Autodesk Inventor part; units mm, degrees
(part 2 of 6)
  line L449 (30.3134, 44.4626) -> (30.5187, 44.7625) construction
  line L450 (30.5187, 44.7625) -> (30.9923, 45.236) construction
  line L451 (30.9923, 45.236) -> (31.2921, 45.4412) construction
  line L452 (31.2921, 45.4412) -> (31.9491, 45.7133) construction
  line L453 (31.9491, 45.7133) -> (32.3063, 45.7803) construction
  line L454 (32.3063, 45.7803) -> (32.9761, 45.7803) construction
  line L455 (32.9761, 45.7803) -> (33.3332, 45.7133) construction
  line L456 (33.3332, 45.7133) -> (33.9902, 45.4412) construction
  line L457 (33.9902, 45.4412) -> (34.2901, 45.236) construction
  line L458 (34.2901, 45.236) -> (34.7637, 44.7625) construction
  line L459 (34.7637, 44.7625) -> (34.969, 44.4626) construction
  line L460 (34.969, 44.4626) -> (35.2413, 43.8054) construction
  line L461 (35.2413, 43.8054) -> (35.3082, 43.4482) construction
  line L462 (35.3082, 43.4482) -> (35.3082, 42.7784) construction
  line L463 (35.3082, 42.7784) -> (35.2413, 42.4212) construction
  line L464 (35.2413, 42.4212) -> (34.969, 41.764) construction
  line L465 (34.969, 41.764) -> (34.7638, 41.4641) construction
  line L466 (34.7638, 41.4641) -> (34.2901, 40.9905) construction
  line L467 (34.2901, 40.9905) -> (33.9903, 40.7853) construction
  line L468 (33.9903, 40.7853) -> (33.3332, 40.5132) construction
  line L469 (33.3332, 40.5132) -> (32.976, 40.4463) construction
  line L470 (32.976, 40.4463) -> (32.6412, 40.4463) construction
  circle A90 centre (-16.6963, 38.4758) radius 1.25
  circle A91 centre (15.3037, 6.4758) radius 1.25
  circle A92 centre (15.3037, 38.4758) radius 1.25
  circle A93 centre (-16.6963, 6.4758) radius 1.25
  arc A94 (39.458, -65.8975) -> (33.108, -59.5475) centre (33.108, -65.8975) ccw
  line L471 (33.108, -59.5475) -> (31.785, -59.5475)
  arc A95 (26.4124, -59.0625) -> (31.785, -59.5475) centre (31.785, -29.5475) ccw
  arc A96 (26.4124, -59.0625) -> (21.0398, -58.5775) centre (21.0398, -88.5775) ccw
  line L472 (21.0398, -58.5775) -> (-15.8645, -58.5775)
  arc A97 (-15.8645, -56.5775) -> (-15.8645, -58.5775) centre (-15.8645, -57.5775) ccw
  line L473 (-15.8645, -56.5775) -> (23.218, -56.5775)
  arc A98 (23.218, -56.5775) -> (23.218, -54.5775) centre (23.218, -55.5775) ccw
  line L474 (23.218, -54.5775) -> (-15.8645, -54.5775)
  arc A99 (-15.8645, -52.5775) -> (-15.8645, -54.5775) centre (-15.8645, -53.5775) ccw
  line L475 (-15.8645, -52.5775) -> (23.218, -52.5775)
  arc A100 (23.218, -52.5775) -> (23.218, -50.5775) centre (23.218, -51.5775) ccw
  line L476 (23.218, -50.5775) -> (-15.8645, -50.5775)
  arc A101 (-15.8645, -48.5775) -> (-15.8645, -50.5775) centre (-15.8645, -49.5775) ccw
  line L477 (-15.8645, -48.5775) -> (23.218, -48.5775)
  arc A102 (23.218, -48.5775) -> (23.218, -46.5775) centre (23.218, -47.5775) ccw
  line L478 (23.218, -46.5775) -> (-15.8645, -46.5775)
  arc A103 (-15.8645, -44.5775) -> (-15.8645, -46.5775) centre (-15.8645, -45.5775) ccw
  line L479 (-15.8645, -44.5775) -> (23.218, -44.5775)
  arc A104 (23.218, -44.5775) -> (23.218, -42.5775) centre (23.218, -43.5775) ccw
  line L480 (23.218, -42.5775) -> (-15.8645, -42.5775)
  arc A105 (-15.8645, -40.5775) -> (-15.8645, -42.5775) centre (-15.8645, -41.5775) ccw
  line L481 (-15.8645, -40.5775) -> (23.218, -40.5775)
  arc A106 (23.218, -40.5775) -> (23.218, -38.5775) centre (23.218, -39.5775) ccw
  line L482 (23.218, -38.5775) -> (-15.8645, -38.5775)
  arc A107 (-15.8645, -36.5775) -> (-15.8645, -38.5775) centre (-15.8645, -37.5775) ccw
  line L483 (-15.8645, -36.5775) -> (23.218, -36.5775)
  arc A108 (23.218, -36.5775) -> (23.218, -34.5775) centre (23.218, -35.5775) ccw
  line L484 (23.218, -34.5775) -> (-15.8645, -34.5775)
  arc A109 (-15.8645, -32.5775) -> (-15.8645, -34.5775) centre (-15.8645, -33.5775) ccw
  line L485 (-15.8645, -32.5775) -> (21.0398, -32.5775)
  arc A110 (21.0398, -32.5775) -> (26.4124, -32.0925) centre (21.0398, -2.5775) ccw
  arc A111 (31.785, -31.6075) -> (26.4124, -32.0925) centre (31.785, -61.6075) ccw
  line L486 (31.785, -31.6075) -> (33.743, -31.6075)
  arc A112 (33.743, -31.6075) -> (40.093, -25.2575) centre (33.743, -25.2575) ccw
  line L487 (40.093, -25.2575) -> (40.093, -19.225)
  arc A113 (40.093, -19.225) -> (38.5055, -17.6375) centre (38.5055, -19.225) ccw
  line L488 (38.5055, -17.6375) -> (-36.4245, -17.6375)
  arc A114 (-36.4245, -17.6375) -> (-38.012, -19.225) centre (-36.4245, -19.225) ccw
  line L489 (-38.012, -19.225) -> (-38.012, -71.9264)
  arc A115 (-38.012, -71.9264) -> (-36.4245, -73.5139) centre (-36.4245, -71.9264) ccw
  line L490 (-36.4245, -73.5139) -> (37.8705, -73.5139)
  arc A116 (37.8705, -73.5139) -> (39.458, -71.9264) centre (37.8705, -71.9264) ccw
  line L491 (39.458, -71.9264) -> (39.458, -65.8975)
  spline S16 degree 3 poles (-31.027, -27.607) (-31.3618, -27.607) (-31.719, -27.5401) (-32.376, -27.2679) (-32.6759, -27.0627) (-33.1495, -26.5892) (-33.3548, -26.2892) (-33.627, -25.6321) (-33.694, -25.2748) (-33.694, -24.6051) (-33.627, -24.2478) (-33.3548, -23.5907) (-33.1495, -23.2907) (-32.6759, -22.8172) (-32.376, -22.612) (-31.719, -22.3399) (-31.3618, -22.273) (-30.6921, -22.273) (-30.3349, -22.3399) (-29.6779, -22.612) (-29.3781, -22.8172) (-28.9044, -23.2907) (-28.6991, -23.5907) (-28.4269, -24.2478) (-28.36, -24.6051) (-28.36, -25.2748) (-28.4269, -25.6321) (-28.6991, -26.2892) (-28.9044, -26.5892) (-29.378, -27.0627) (-29.6779, -27.2679) (-30.3349, -27.5401) (-30.6921, -27.607) (-31.027, -27.607) knots -1.607821 -1.607821 -1.607821 -1.607821 -1.507362 -1.507362 -1.406903 -1.406903 -1.30639 -1.30639 -1.205878 -1.205878 -1.105355 -1.105355 -1.004831 -1.004831 -0.904371 -0.904371 -0.803911 -0.803911 -0.70345 -0.70345 -0.60299 -0.60299 -0.502467 -0.502467 -0.401943 -0.401943 -0.301431 -0.301431 -0.200918 -0.200918 -0.100459 -0.100459 0 0 0 0
  line L492 (-31.027, -27.607) -> (-31.3618, -27.607) construction
  line L493 (-31.3618, -27.607) -> (-31.719, -27.5401) construction
  line L494 (-31.719, -27.5401) -> (-32.376, -27.2679) construction
  line L495 (-32.376, -27.2679) -> (-32.6759, -27.0627) construction
  line L496 (-32.6759, -27.0627) -> (-33.1495, -26.5892) construction
  line L497 (-33.1495, -26.5892) -> (-33.3548, -26.2892) construction
  line L498 (-33.3548, -26.2892) -> (-33.627, -25.6321) construction
  line L499 (-33.627, -25.6321) -> (-33.694, -25.2748) construction
  line L500 (-33.694, -25.2748) -> (-33.694, -24.6051) construction
  line L501 (-33.694, -24.6051) -> (-33.627, -24.2478) construction
  line L502 (-33.627, -24.2478) -> (-33.3548, -23.5907) construction
  line L503 (-33.3548, -23.5907) -> (-33.1495, -23.2907) construction
  line L504 (-33.1495, -23.2907) -> (-32.6759, -22.8172) construction
  line L505 (-32.6759, -22.8172) -> (-32.376, -22.612) construction
  line L506 (-32.376, -22.612) -> (-31.719, -22.3399) construction
  line L507 (-31.719, -22.3399) -> (-31.3618, -22.273) construction
  line L508 (-31.3618, -22.273) -> (-30.6921, -22.273) construction
  line L509 (-30.6921, -22.273) -> (-30.3349, -22.3399) construction
  line L510 (-30.3349, -22.3399) -> (-29.6779, -22.612) construction
  line L511 (-29.6779, -22.612) -> (-29.3781, -22.8172) construction
  line L512 (-29.3781, -22.8172) -> (-28.9044, -23.2907) construction
  line L513 (-28.9044, -23.2907) -> (-28.6991, -23.5907) construction
  line L514 (-28.6991, -23.5907) -> (-28.4269, -24.2478) construction
  line L515 (-28.4269, -24.2478) -> (-28.36, -24.6051) construction
  line L516 (-28.36, -24.6051) -> (-28.36, -25.2748) construction
  line L517 (-28.36, -25.2748) -> (-28.4269, -25.6321) construction
  line L518 (-28.4269, -25.6321) -> (-28.6991, -26.2892) construction
  line L519 (-28.6991, -26.2892) -> (-28.9044, -26.5892) construction
  line L520 (-28.9044, -26.5892) -> (-29.378, -27.0627) construction
  line L521 (-29.378, -27.0627) -> (-29.6779, -27.2679) construction
  line L522 (-29.6779, -27.2679) -> (-30.3349, -27.5401) construction
  line L523 (-30.3349, -27.5401) -> (-30.6921, -27.607) construction
  line L524 (-30.6921, -27.607) -> (-31.027, -27.607) construction
  spline S17 degree 3 poles (-31.027, -68.882) (-31.3618, -68.882) (-31.719, -68.8151) (-32.376, -68.5429) (-32.6759, -68.3377) (-33.1495, -67.8642) (-33.3548, -67.5643) (-33.627, -66.9071) (-33.694, -66.5499) (-33.694, -65.8801) (-33.627, -65.5229) (-33.3548, -64.8657) (-33.1495, -64.5658) (-32.6759, -64.0922) (-32.376, -63.887) (-31.719, -63.6149) (-31.3618, -63.548) (-30.6921, -63.548) (-30.3349, -63.6149) (-29.6779, -63.887) (-29.378, -64.0922) (-28.9044, -64.5658) (-28.6991, -64.8657) (-28.4269, -65.5229) (-28.36, -65.8801) (-28.36, -66.5499) (-28.4269, -66.9071) (-28.6991, -67.5643) (-28.9044, -67.8642) (-29.3781, -68.3377) (-29.6779, -68.5429) (-30.3349, -68.8151) (-30.6921, -68.882) (-31.027, -68.882) knots -1.607821 -1.607821 -1.607821 -1.607821 -1.507361 -1.507361 -1.406901 -1.406901 -1.306377 -1.306377 -1.205854 -1.205854 -1.105342 -1.105342 -1.004829 -1.004829 -0.90437 -0.90437 -0.803911 -0.803911 -0.703451 -0.703451 -0.602992 -0.602992 -0.50248 -0.50248 -0.401967 -0.401967 -0.301444 -0.301444 -0.200921 -0.200921 -0.10046 -0.10046 0 0 0 0
  line L525 (-31.027, -68.882) -> (-31.3618, -68.882) construction
  line L526 (-31.3618, -68.882) -> (-31.719, -68.8151) construction
  line L527 (-31.719, -68.8151) -> (-32.376, -68.5429) construction
  line L528 (-32.376, -68.5429) -> (-32.6759, -68.3377) construction
  line L529 (-32.6759, -68.3377) -> (-33.1495, -67.8642) construction
  line L530 (-33.1495, -67.8642) -> (-33.3548, -67.5643) construction
  line L531 (-33.3548, -67.5643) -> (-33.627, -66.9071) construction
  line L532 (-33.627, -66.9071) -> (-33.694, -66.5499) construction
  line L533 (-33.694, -66.5499) -> (-33.694, -65.8801) construction
  line L534 (-33.694, -65.8801) -> (-33.627, -65.5229) construction
  line L535 (-33.627, -65.5229) -> (-33.3548, -64.8657) construction
  line L536 (-33.3548, -64.8657) -> (-33.1495, -64.5658) construction
  line L537 (-33.1495, -64.5658) -> (-32.6759, -64.0922) construction
  line L538 (-32.6759, -64.0922) -> (-32.376, -63.887) construction
  line L539 (-32.376, -63.887) -> (-31.719, -63.6149) construction
  line L540 (-31.719, -63.6149) -> (-31.3618, -63.548) construction
  line L541 (-31.3618, -63.548) -> (-30.6921, -63.548) construction
  line L542 (-30.6921, -63.548) -> (-30.3349, -63.6149) construction
  line L543 (-30.3349, -63.6149) -> (-29.6779, -63.887) construction
  line L544 (-29.6779, -63.887) -> (-29.378, -64.0922) construction
  line L545 (-29.378, -64.0922) -> (-28.9044, -64.5658) construction
  line L546 (-28.9044, -64.5658) -> (-28.6991, -64.8657) construction
  line L547 (-28.6991, -64.8657) -> (-28.4269, -65.5229) construction
  line L548 (-28.4269, -65.5229) -> (-28.36, -65.8801) construction
  line L549 (-28.36, -65.8801) -> (-28.36, -66.5499) construction
  line L550 (-28.36, -66.5499) -> (-28.4269, -66.9071) construction
  line L551 (-28.4269, -66.9071) -> (-28.6991, -67.5643) construction
  line L552 (-28.6991, -67.5643) -> (-28.9044, -67.8642) construction
  line L553 (-28.9044, -67.8642) -> (-29.3781, -68.3377) construction
  line L554 (-29.3781, -68.3377) -> (-29.6779, -68.5429) construction
  line L555 (-29.6779, -68.5429) -> (-30.3349, -68.8151) construction
  line L556 (-30.3349, -68.8151) -> (-30.6921, -68.882) construction
  line L557 (-30.6921, -68.882) -> (-31.027, -68.882) construction
  spline S18 degree 3 poles (32.473, -68.882) (32.1382, -68.882) (31.781, -68.8151) (31.124, -68.5429) (30.8241, -68.3377) (30.3505, -67.8642) (30.1452, -67.5643) (29.873, -66.9071) (29.806, -66.5499) (29.806, -65.8801) (29.873, -65.5229) (30.1452, -64.8657) (30.3505, -64.5658) (30.8241, -64.0922) (31.124, -63.887) (31.781, -63.6149) (32.1382, -63.548) (32.8079, -63.548) (33.1651, -63.6149) (33.8221, -63.887) (34.122, -64.0922) (34.5956, -64.5658) (34.8009, -64.8657) (35.0731, -65.5229) (35.14, -65.8801) (35.14, -66.5499) (35.0731, -66.9071) (34.8009, -67.5643) (34.5956, -67.8642) (34.1219, -68.3377) (33.8221, -68.5429) (33.1651, -68.8151) (32.8079, -68.882) (32.473, -68.882) knots -1.607821 -1.607821 -1.607821 -1.607821 -1.507361 -1.507361 -1.406901 -1.406901 -1.306377 -1.306377 -1.205854 -1.205854 -1.105342 -1.105342 -1.004829 -1.004829 -0.90437 -0.90437 -0.803911 -0.803911 -0.703451 -0.703451 -0.602992 -0.602992 -0.50248 -0.50248 -0.401967 -0.401967 -0.301444 -0.301444 -0.200921 -0.200921 -0.10046 -0.10046 0 0 0 0
  line L558 (32.473, -68.882) -> (32.1382, -68.882) construction
  line L559 (32.1382, -68.882) -> (31.781, -68.8151) construction
  line L560 (31.781, -68.8151) -> (31.124, -68.5429) construction
  line L561 (31.124, -68.5429) -> (30.8241, -68.3377) construction
  line L562 (30.8241, -68.3377) -> (30.3505, -67.8642) construction
  line L563 (30.3505, -67.8642) -> (30.1452, -67.5643) construction
  line L564 (30.1452, -67.5643) -> (29.873, -66.9071) construction
  line L565 (29.873, -66.9071) -> (29.806, -66.5499) construction
  line L566 (29.806, -66.5499) -> (29.806, -65.8801) construction
  line L567 (29.806, -65.8801) -> (29.873, -65.5229) construction
  line L568 (29.873, -65.5229) -> (30.1452, -64.8657) construction
  line L569 (30.1452, -64.8657) -> (30.3505, -64.5658) construction
  line L570 (30.3505, -64.5658) -> (30.8241, -64.0922) construction
  line L571 (30.8241, -64.0922) -> (31.124, -63.887) construction
  line L572 (31.124, -63.887) -> (31.781, -63.6149) construction
  line L573 (31.781, -63.6149) -> (32.1382, -63.548) construction
  line L574 (32.1382, -63.548) -> (32.8079, -63.548) construction
  line L575 (32.8079, -63.548) -> (33.1651, -63.6149) construction
  line L576 (33.1651, -63.6149) -> (33.8221, -63.887) construction
  line L577 (33.8221, -63.887) -> (34.122, -64.0922) construction
  line L578 (34.122, -64.0922) -> (34.5956, -64.5658) construction
  line L579 (34.5956, -64.5658) -> (34.8009, -64.8657) construction
  line L580 (34.8009, -64.8657) -> (35.0731, -65.5229) construction
  line L581 (35.0731, -65.5229) -> (35.14, -65.8801) construction
  line L582 (35.14, -65.8801) -> (35.14, -66.5499) construction
  line L583 (35.14, -66.5499) -> (35.0731, -66.9071) construction
  line L584 (35.0731, -66.9071) -> (34.8009, -67.5643) construction
  line L585 (34.8009, -67.5643) -> (34.5956, -67.8642) construction
  line L586 (34.5956, -67.8642) -> (34.1219, -68.3377) construction
  line L587 (34.1219, -68.3377) -> (33.8221, -68.5429) construction
  line L588 (33.8221, -68.5429) -> (33.1651, -68.8151) construction
  line L589 (33.1651, -68.8151) -> (32.8079, -68.882) construction
  line L590 (32.8079, -68.882) -> (32.473, -68.882) construction
  spline S19 degree 3 poles (32.473, -27.607) (32.1382, -27.607) (31.781, -27.5401) (31.124, -27.2679) (30.8241, -27.0627) (30.3505, -26.5892) (30.1452, -26.2892) (29.873, -25.6321) (29.806, -25.2748) (29.806, -24.6051) (29.873, -24.2478) (30.1452, -23.5907) (30.3505, -23.2907) (30.8241, -22.8172) (31.124, -22.612) (31.781, -22.3399) (32.1382, -22.273) (32.8079, -22.273) (33.1651, -22.3399) (33.8221, -22.612) (34.1219, -22.8172) (34.5956, -23.2907) (34.8009, -23.5907) (35.0731, -24.2478) (35.14, -24.6051) (35.14, -25.2748) (35.0731, -25.6321) (34.8009, -26.2892) (34.5956, -26.5892) (34.122, -27.0627) (33.8221, -27.2679) (33.1651, -27.5401) (32.8079, -27.607) (32.473, -27.607) knots -1.607821 -1.607821 -1.607821 -1.607821 -1.507362 -1.507362 -1.406903 -1.406903 -1.30639 -1.30639 -1.205878 -1.205878 -1.105355 -1.105355 -1.004831 -1.004831 -0.904371 -0.904371 -0.803911 -0.803911 -0.70345 -0.70345 -0.60299 -0.60299 -0.502467 -0.502467 -0.401943 -0.401943 -0.301431 -0.301431 -0.200918 -0.200918 -0.100459 -0.100459 0 0 0 0
  line L591 (32.473, -27.607) -> (32.1382, -27.607) construction
  line L592 (32.1382, -27.607) -> (31.781, -27.5401) construction
  line L593 (31.781, -27.5401) -> (31.124, -27.2679) construction
  line L594 (31.124, -27.2679) -> (30.8241, -27.0627) construction
  line L595 (30.8241, -27.0627) -> (30.3505, -26.5892) construction
  line L596 (30.3505, -26.5892) -> (30.1452, -26.2892) construction
  line L597 (30.1452, -26.2892) -> (29.873, -25.6321) construction
  line L598 (29.873, -25.6321) -> (29.806, -25.2748) construction
  line L599 (29.806, -25.2748) -> (29.806, -24.6051) construction
  line L600 (29.806, -24.6051) -> (29.873, -24.2478) construction
  line L601 (29.873, -24.2478) -> (30.1452, -23.5907) construction
  line L602 (30.1452, -23.5907) -> (30.3505, -23.2907) construction
  line L603 (30.3505, -23.2907) -> (30.8241, -22.8172) construction
  line L604 (30.8241, -22.8172) -> (31.124, -22.612) construction
  line L605 (31.124, -22.612) -> (31.781, -22.3399) construction
  line L606 (31.781, -22.3399) -> (32.1382, -22.273) construction
  line L607 (32.1382, -22.273) -> (32.8079, -22.273) construction
  line L608 (32.8079, -22.273) -> (33.1651, -22.3399) construction
  line L609 (33.1651, -22.3399) -> (33.8221, -22.612) construction
  line L610 (33.8221, -22.612) -> (34.1219, -22.8172) construction
  line L611 (34.1219, -22.8172) -> (34.5956, -23.2907) construction
  line L612 (34.5956, -23.2907) -> (34.8009, -23.5907) construction
  line L613 (34.8009, -23.5907) -> (35.0731, -24.2478) construction
  line L614 (35.0731, -24.2478) -> (35.14, -24.6051) construction
  line L615 (35.14, -24.6051) -> (35.14, -25.2748) construction
  line L616 (35.14, -25.2748) -> (35.0731, -25.6321) construction
  line L617 (35.0731, -25.6321) -> (34.8009, -26.2892) construction
  line L618 (34.8009, -26.2892) -> (34.5956, -26.5892) construction
  line L619 (34.5956, -26.5892) -> (34.122, -27.0627) construction
  line L620 (34.122, -27.0627) -> (33.8221, -27.2679) construction
  line L621 (33.8221, -27.2679) -> (33.1651, -27.5401) construction
  line L622 (33.1651, -27.5401) -> (32.8079, -27.607) construction
  line L623 (32.8079, -27.607) -> (32.473, -27.607) construction
  circle A117 centre (-16.8645, -29.5775) radius 1.25
  circle A118 centre (15.1355, -61.5775) radius 1.25
  circle A119 centre (15.1355, -29.5775) radius 1.25
  circle A120 centre (-16.8645, -61.5775) radius 1.25
  arc A121 (-65.5764, 238.6382) -> (-63.5764, 238.6382) centre (-64.5764, 238.6382) ccw
  arc A122 (-59.0914, 280.9151) -> (-59.5764, 275.5425) centre (-29.5764, 275.5425) ccw
  circle A123 centre (-56.5764, 237.6382) radius 1.25
  arc A124 (-77.5764, 238.6382) -> (-75.5764, 238.6382) centre (-76.5764, 238.6382) ccw
  arc A125 (-85.5764, 238.6382) -> (-83.5764, 238.6382) centre (-84.5764, 238.6382) ccw
  line L624 (-59.5764, 275.5425) -> (-59.5764, 238.6382)
  line L625 (-63.5764, 277.7207) -> (-63.5764, 238.6382)
  line L626 (-65.5764, 238.6382) -> (-65.5764, 277.7207)
  line L627 (-61.5764, 238.6382) -> (-61.5764, 277.7207)
  line L628 (-67.5764, 277.7207) -> (-67.5764, 238.6382)
  line L629 (-71.5764, 277.7207) -> (-71.5764, 238.6382)
  line L630 (-73.5764, 238.6382) -> (-73.5764, 277.7207)
  line L631 (-75.5764, 277.7207) -> (-75.5764, 238.6382)
  line L632 (-77.5764, 238.6382) -> (-77.5764, 277.7207)
  line L633 (-79.5764, 277.7207) -> (-79.5764, 238.6382)
  line L634 (-85.5764, 238.6382) -> (-85.5764, 275.5425)
  line L635 (-81.5764, 238.6382) -> (-81.5764, 277.7207)
  line L636 (-83.5764, 277.7207) -> (-83.5764, 238.6382)
  arc A126 (-59.0914, 280.9151) -> (-58.6064, 286.2877) centre (-88.6064, 286.2877) ccw
  line L637 (-58.6064, 287.6107) -> (-58.6064, 286.2877)
  line L638 (-44.64, 218.0782) -> (-44.64, 292.3732)
  line L639 (-100.5164, 293.0082) -> (-100.5164, 218.0782)
  line L640 (-69.5764, 238.6382) -> (-69.5764, 277.7207)
  arc A127 (-73.5764, 238.6382) -> (-71.5764, 238.6382) centre (-72.5764, 238.6382) ccw
  arc A128 (-65.5764, 277.7207) -> (-67.5764, 277.7207) centre (-66.5764, 277.7207) ccw
  arc A129 (-73.5764, 277.7207) -> (-75.5764, 277.7207) centre (-74.5764, 277.7207) ccw
  arc A130 (-61.5764, 277.7207) -> (-63.5764, 277.7207) centre (-62.5764, 277.7207) ccw
  circle A131 centre (-56.5764, 269.6382) radius 1.25
  line L641 (-91.5647, 284.8531) -> (-91.8647, 284.6478) construction
  spline S20 degree 3 poles (-90.5469, 286.9757) (-90.5469, 286.6408) (-90.6138, 286.2837) (-90.886, 285.6266) (-91.0912, 285.3268) (-91.5647, 284.8531) (-91.8647, 284.6478) (-92.5218, 284.3756) (-92.879, 284.3087) (-93.5488, 284.3087) (-93.906, 284.3756) (-94.5632, 284.6479) (-94.8631, 284.8532) (-95.3367, 285.3268) (-95.5419, 285.6266) (-95.814, 286.2837) (-95.8809, 286.6408) (-95.8809, 287.3106) (-95.814, 287.6677) (-95.5419, 288.3248) (-95.3367, 288.6246) (-94.8631, 289.0982) (-94.5632, 289.3035) (-93.906, 289.5758) (-93.5488, 289.6427) (-92.879, 289.6427) (-92.5218, 289.5758) (-91.8647, 289.3036) (-91.5647, 289.0983) (-91.0912, 288.6246) (-90.886, 288.3248) (-90.6138, 287.6677) (-90.5469, 287.3106) (-90.5469, 286.9757) knots -1.607821 -1.607821 -1.607821 -1.607821 -1.507362 -1.507362 -1.406903 -1.406903 -1.30639 -1.30639 -1.205878 -1.205878 -1.105355 -1.105355 -1.004831 -1.004831 -0.904371 -0.904371 -0.803911 -0.803911 -0.70345 -0.70345 -0.60299 -0.60299 -0.502467 -0.502467 -0.401943 -0.401943 -0.301431 -0.301431 -0.200918 -0.200918 -0.100459 -0.100459 0 0 0 0
  line L642 (-90.5469, 286.9757) -> (-90.5469, 286.6408) construction
  line L643 (-90.5469, 286.6408) -> (-90.6138, 286.2837) construction
  line L644 (-90.6138, 286.2837) -> (-90.886, 285.6266) construction
  line L645 (-90.886, 285.6266) -> (-91.0912, 285.3268) construction
  line L646 (-91.0912, 285.3268) -> (-91.5647, 284.8531) construction
  line L647 (-91.8647, 284.6478) -> (-92.5218, 284.3756) construction
  line L648 (-92.5218, 284.3756) -> (-92.879, 284.3087) construction
  line L649 (-92.879, 284.3087) -> (-93.5488, 284.3087) construction
  line L650 (-93.5488, 284.3087) -> (-93.906, 284.3756) construction
  line L651 (-93.906, 284.3756) -> (-94.5632, 284.6479) construction
  line L652 (-94.5632, 284.6479) -> (-94.8631, 284.8532) construction
  line L653 (-94.8631, 284.8532) -> (-95.3367, 285.3268) construction
  line L654 (-95.3367, 285.3268) -> (-95.5419, 285.6266) construction
  line L655 (-95.5419, 285.6266) -> (-95.814, 286.2837) construction
  line L656 (-95.814, 286.2837) -> (-95.8809, 286.6408) construction
  line L657 (-95.8809, 286.6408) -> (-95.8809, 287.3106) construction
  line L658 (-95.8809, 287.3106) -> (-95.814, 287.6677) construction
  line L659 (-95.814, 287.6677) -> (-95.5419, 288.3248) construction
  line L660 (-95.5419, 288.3248) -> (-95.3367, 288.6246) construction
  line L661 (-95.3367, 288.6246) -> (-94.8631, 289.0982) construction
  line L662 (-94.8631, 289.0982) -> (-94.5632, 289.3035) construction
  line L663 (-94.5632, 289.3035) -> (-93.906, 289.5758) construction
  line L664 (-93.906, 289.5758) -> (-93.5488, 289.6427) construction
  line L665 (-93.5488, 289.6427) -> (-92.879, 289.6427) construction
  line L666 (-92.879, 289.6427) -> (-92.5218, 289.5758) construction
  line L667 (-92.5218, 289.5758) -> (-91.8647, 289.3036) construction
  line L668 (-91.8647, 289.3036) -> (-91.5647, 289.0983) construction
  line L669 (-91.5647, 289.0983) -> (-91.0912, 288.6246) construction
  line L670 (-91.0912, 288.6246) -> (-90.886, 288.3248) construction
  line L671 (-90.886, 288.3248) -> (-90.6138, 287.6677) construction
  line L672 (-90.6138, 287.6677) -> (-90.5469, 287.3106) construction
  line L673 (-90.5469, 287.3106) -> (-90.5469, 286.9757) construction
  circle A132 centre (-88.5764, 269.6382) radius 1.25
  arc A133 (-85.5764, 275.5425) -> (-86.0614, 280.9151) centre (-115.5764, 275.5425) ccw
  arc A134 (-86.5464, 286.2877) -> (-86.0614, 280.9151) centre (-56.5464, 286.2877) ccw
  arc A135 (-81.5764, 277.7207) -> (-83.5764, 277.7207) centre (-82.5764, 277.7207) ccw
  arc A136 (-86.5464, 288.2457) -> (-92.8964, 294.5957) centre (-92.8964, 288.2457) ccw
  line L674 (-92.8964, 294.5957) -> (-98.9289, 294.5957)
  arc A137 (-98.9289, 294.5957) -> (-100.5164, 293.0082) centre (-98.9289, 293.0082) ccw
  line L675 (-86.5464, 286.2877) -> (-86.5464, 288.2457)
  arc A138 (-52.2564, 293.9607) -> (-58.6064, 287.6107) centre (-52.2564, 287.6107) ccw
  arc A139 (-69.5764, 277.7207) -> (-71.5764, 277.7207) centre (-70.5764, 277.7207) ccw
  arc A140 (-77.5764, 277.7207) -> (-79.5764, 277.7207) centre (-78.5764, 277.7207) ccw
  line L676 (-49.2719, 286.6408) -> (-49.3388, 286.2837) construction
  spline S21 degree 3 poles (-49.2719, 286.9757) (-49.2719, 286.6408) (-49.3388, 286.2837) (-49.6109, 285.6266) (-49.8161, 285.3268) (-50.2897, 284.8532) (-50.5896, 284.6479) (-51.2468, 284.3756) (-51.604, 284.3087) (-52.2738, 284.3087) (-52.631, 284.3756) (-53.2881, 284.6478) (-53.5881, 284.8531) (-54.0616, 285.3268) (-54.2668, 285.6266) (-54.539, 286.2837) (-54.6059, 286.6408) (-54.6059, 287.3106) (-54.539, 287.6677) (-54.2668, 288.3248) (-54.0616, 288.6246) (-53.5881, 289.0983) (-53.2881, 289.3036) (-52.631, 289.5758) (-52.2738, 289.6427) (-51.604, 289.6427) (-51.2468, 289.5758) (-50.5896, 289.3035) (-50.2897, 289.0982) (-49.8161, 288.6246) (-49.6109, 288.3248) (-49.3388, 287.6677) (-49.2719, 287.3106) (-49.2719, 286.9757) knots -1.607821 -1.607821 -1.607821 -1.607821 -1.507361 -1.507361 -1.406901 -1.406901 -1.306377 -1.306377 -1.205854 -1.205854 -1.105342 -1.105342 -1.004829 -1.004829 -0.90437 -0.90437 -0.803911 -0.803911 -0.703451 -0.703451 -0.602992 -0.602992 -0.50248 -0.50248 -0.401967 -0.401967 -0.301444 -0.301444 -0.200921 -0.200921 -0.10046 -0.10046 0 0 0 0
  line L677 (-49.2719, 286.9757) -> (-49.2719, 286.6408) construction
  line L678 (-49.3388, 286.2837) -> (-49.6109, 285.6266) construction
  line L679 (-49.6109, 285.6266) -> (-49.8161, 285.3268) construction
  line L680 (-49.8161, 285.3268) -> (-50.2897, 284.8532) construction
  line L681 (-50.2897, 284.8532) -> (-50.5896, 284.6479) construction
  line L682 (-50.5896, 284.6479) -> (-51.2468, 284.3756) construction
  line L683 (-51.2468, 284.3756) -> (-51.604, 284.3087) construction
  line L684 (-51.604, 284.3087) -> (-52.2738, 284.3087) construction
  line L685 (-52.2738, 284.3087) -> (-52.631, 284.3756) construction
  line L686 (-52.631, 284.3756) -> (-53.2881, 284.6478) construction
  line L687 (-53.2881, 284.6478) -> (-53.5881, 284.8531) construction
  line L688 (-53.5881, 284.8531) -> (-54.0616, 285.3268) construction
  line L689 (-54.0616, 285.3268) -> (-54.2668, 285.6266) construction
  line L690 (-54.2668, 285.6266) -> (-54.539, 286.2837) construction
  line L691 (-54.539, 286.2837) -> (-54.6059, 286.6408) construction
  line L692 (-54.6059, 286.6408) -> (-54.6059, 287.3106) construction
  line L693 (-54.6059, 287.3106) -> (-54.539, 287.6677) construction
  line L694 (-54.539, 287.6677) -> (-54.2668, 288.3248) construction
  line L695 (-54.2668, 288.3248) -> (-54.0616, 288.6246) construction
  line L696 (-54.0616, 288.6246) -> (-53.5881, 289.0983) construction
  line L697 (-53.5881, 289.0983) -> (-53.2881, 289.3036) construction
  line L698 (-53.2881, 289.3036) -> (-52.631, 289.5758) construction
  line L699 (-52.631, 289.5758) -> (-52.2738, 289.6427) construction
  line L700 (-52.2738, 289.6427) -> (-51.604, 289.6427) construction
  line L701 (-51.604, 289.6427) -> (-51.2468, 289.5758) construction
  line L702 (-51.2468, 289.5758) -> (-50.5896, 289.3035) construction
  line L703 (-50.5896, 289.3035) -> (-50.2897, 289.0982) construction
  line L704 (-50.2897, 289.0982) -> (-49.8161, 288.6246) construction
  line L705 (-49.8161, 288.6246) -> (-49.6109, 288.3248) construction
  line L706 (-49.6109, 288.3248) -> (-49.3388, 287.6677) construction
  line L707 (-49.3388, 287.6677) -> (-49.2719, 287.3106) construction
  line L708 (-49.2719, 287.3106) -> (-49.2719, 286.9757) construction
  arc A141 (-44.64, 292.3732) -> (-46.2275, 293.9607) centre (-46.2275, 292.3732) ccw
  line L709 (-46.2275, 293.9607) -> (-52.2564, 293.9607)
  arc A142 (-46.2275, 216.4907) -> (-44.64, 218.0782) centre (-46.2275, 218.0782) ccw
  line L710 (-49.3388, 222.7837) -> (-49.6109, 222.1266) construction
  spline S22 degree 3 poles (-49.2719, 223.4757) (-49.2719, 223.1408) (-49.3388, 222.7837) (-49.6109, 222.1266) (-49.8161, 221.8268) (-50.2897, 221.3532) (-50.5896, 221.1479) (-51.2468, 220.8756) (-51.604, 220.8087) (-52.2738, 220.8087) (-52.631, 220.8756) (-53.2881, 221.1478) (-53.5881, 221.3531) (-54.0616, 221.8268) (-54.2668, 222.1266) (-54.539, 222.7837) (-54.6059, 223.1408) (-54.6059, 223.8106) (-54.539, 224.1677) (-54.2668, 224.8248) (-54.0616, 225.1246) (-53.5881, 225.5983) (-53.2881, 225.8036) (-52.631, 226.0758) (-52.2738, 226.1427) (-51.604, 226.1427) (-51.2468, 226.0758) (-50.5896, 225.8035) (-50.2897, 225.5982) (-49.8161, 225.1246) (-49.6109, 224.8248) (-49.3388, 224.1677) (-49.2719, 223.8106) (-49.2719, 223.4757) knots -1.607821 -1.607821 -1.607821 -1.607821 -1.507361 -1.507361 -1.406901 -1.406901 -1.306377 -1.306377 -1.205854 -1.205854 -1.105342 -1.105342 -1.004829 -1.004829 -0.90437 -0.90437 -0.803911 -0.803911 -0.703451 -0.703451 -0.602992 -0.602992 -0.50248 -0.50248 -0.401967 -0.401967 -0.301444 -0.301444 -0.200921 -0.200921 -0.10046 -0.10046 0 0 0 0
  line L711 (-49.2719, 223.4757) -> (-49.2719, 223.1408) construction
  line L712 (-49.2719, 223.1408) -> (-49.3388, 222.7837) construction
  line L713 (-49.6109, 222.1266) -> (-49.8161, 221.8268) construction
  line L714 (-49.8161, 221.8268) -> (-50.2897, 221.3532) construction
  line L715 (-50.2897, 221.3532) -> (-50.5896, 221.1479) construction
  line L716 (-50.5896, 221.1479) -> (-51.2468, 220.8756) construction
  line L717 (-51.2468, 220.8756) -> (-51.604, 220.8087) construction
  line L718 (-51.604, 220.8087) -> (-52.2738, 220.8087) construction
  line L719 (-52.2738, 220.8087) -> (-52.631, 220.8756) construction
  line L720 (-52.631, 220.8756) -> (-53.2881, 221.1478) construction
  line L721 (-53.2881, 221.1478) -> (-53.5881, 221.3531) construction
  line L722 (-53.5881, 221.3531) -> (-54.0616, 221.8268) construction
  line L723 (-54.0616, 221.8268) -> (-54.2668, 222.1266) construction
  line L724 (-54.2668, 222.1266) -> (-54.539, 222.7837) construction
  line L725 (-54.539, 222.7837) -> (-54.6059, 223.1408) construction
  line L726 (-54.6059, 223.1408) -> (-54.6059, 223.8106) construction
  line L727 (-54.6059, 223.8106) -> (-54.539, 224.1677) construction
  line L728 (-54.539, 224.1677) -> (-54.2668, 224.8248) construction
  line L729 (-54.2668, 224.8248) -> (-54.0616, 225.1246) construction
  line L730 (-54.0616, 225.1246) -> (-53.5881, 225.5983) construction
  line L731 (-53.5881, 225.5983) -> (-53.2881, 225.8036) construction
  line L732 (-53.2881, 225.8036) -> (-52.631, 226.0758) construction
  line L733 (-52.631, 226.0758) -> (-52.2738, 226.1427) construction
  line L734 (-52.2738, 226.1427) -> (-51.604, 226.1427) construction
  line L735 (-51.604, 226.1427) -> (-51.2468, 226.0758) construction
  line L736 (-51.2468, 226.0758) -> (-50.5896, 225.8035) construction
  line L737 (-50.5896, 225.8035) -> (-50.2897, 225.5982) construction
  line L738 (-50.2897, 225.5982) -> (-49.8161, 225.1246) construction
  line L739 (-49.8161, 225.1246) -> (-49.6109, 224.8248) construction
  line L740 (-49.6109, 224.8248) -> (-49.3388, 224.1677) construction
  line L741 (-49.3388, 224.1677) -> (-49.2719, 223.8106) construction
  line L742 (-49.2719, 223.8106) -> (-49.2719, 223.4757) construction
  arc A143 (-69.5764, 238.6382) -> (-67.5764, 238.6382) centre (-68.5764, 238.6382) ccw
  arc A144 (-61.5764, 238.6382) -> (-59.5764, 238.6382) centre (-60.5764, 238.6382) ccw
  arc A145 (-81.5764, 238.6382) -> (-79.5764, 238.6382) centre (-80.5764, 238.6382) ccw
  line L743 (-91.0912, 225.1246) -> (-90.886, 224.8248) construction
  spline S23 degree 3 poles (-90.5469, 223.4757) (-90.5469, 223.1408) (-90.6138, 222.7837) (-90.886, 222.1266) (-91.0912, 221.8268) (-91.5647, 221.3531) (-91.8647, 221.1478) (-92.5218, 220.8756) (-92.879, 220.8087) (-93.5488, 220.8087) (-93.906, 220.8756) (-94.5632, 221.1479) (-94.8631, 221.3532) (-95.3367, 221.8268) (-95.5419, 222.1266) (-95.814, 222.7837) (-95.8809, 223.1408) (-95.8809, 223.8106) (-95.814, 224.1677) (-95.5419, 224.8248) (-95.3367, 225.1246) (-94.8631, 225.5982) (-94.5632, 225.8035) (-93.906, 226.0758) (-93.5488, 226.1427) (-92.879, 226.1427) (-92.5218, 226.0758) (-91.8647, 225.8036) (-91.5647, 225.5983) (-91.0912, 225.1246) (-90.886, 224.8248) (-90.6138, 224.1677) (-90.5469, 223.8106) (-90.5469, 223.4757) knots -1.607821 -1.607821 -1.607821 -1.607821 -1.507362 -1.507362 -1.406903 -1.406903 -1.30639 -1.30639 -1.205878 -1.205878 -1.105355 -1.105355 -1.004831 -1.004831 -0.904371 -0.904371 -0.803911 -0.803911 -0.70345 -0.70345 -0.60299 -0.60299 -0.502467 -0.502467 -0.401943 -0.401943 -0.301431 -0.301431 -0.200918 -0.200918 -0.100459 -0.100459 0 0 0 0
  line L744 (-90.5469, 223.4757) -> (-90.5469, 223.1408) construction
  line L745 (-90.5469, 223.1408) -> (-90.6138, 222.7837) construction
  line L746 (-90.6138, 222.7837) -> (-90.886, 222.1266) construction
  line L747 (-90.886, 222.1266) -> (-91.0912, 221.8268) construction
  line L748 (-91.0912, 221.8268) -> (-91.5647, 221.3531) construction
  line L749 (-91.5647, 221.3531) -> (-91.8647, 221.1478) construction
  line L750 (-91.8647, 221.1478) -> (-92.5218, 220.8756) construction
  line L751 (-92.5218, 220.8756) -> (-92.879, 220.8087) construction
  line L752 (-92.879, 220.8087) -> (-93.5488, 220.8087) construction
  line L753 (-93.5488, 220.8087) -> (-93.906, 220.8756) construction
  line L754 (-93.906, 220.8756) -> (-94.5632, 221.1479) construction
  line L755 (-94.5632, 221.1479) -> (-94.8631, 221.3532) construction
  line L756 (-94.8631, 221.3532) -> (-95.3367, 221.8268) construction
  line L757 (-95.3367, 221.8268) -> (-95.5419, 222.1266) construction
  line L758 (-95.5419, 222.1266) -> (-95.814, 222.7837) construction
  line L759 (-95.814, 222.7837) -> (-95.8809, 223.1408) construction
  line L760 (-95.8809, 223.1408) -> (-95.8809, 223.8106) construction
  line L761 (-95.8809, 223.8106) -> (-95.814, 224.1677) construction
  line L762 (-95.814, 224.1677) -> (-95.5419, 224.8248) construction
  line L763 (-95.5419, 224.8248) -> (-95.3367, 225.1246) construction
  line L764 (-95.3367, 225.1246) -> (-94.8631, 225.5982) construction
  line L765 (-94.8631, 225.5982) -> (-94.5632, 225.8035) construction
  line L766 (-94.5632, 225.8035) -> (-93.906, 226.0758) construction
  line L767 (-93.906, 226.0758) -> (-93.5488, 226.1427) construction
  line L768 (-93.5488, 226.1427) -> (-92.879, 226.1427) construction
  line L769 (-92.879, 226.1427) -> (-92.5218, 226.0758) construction
  line L770 (-92.5218, 226.0758) -> (-91.8647, 225.8036) construction
  line L771 (-91.8647, 225.8036) -> (-91.5647, 225.5983) construction
  line L772 (-91.5647, 225.5983) -> (-91.0912, 225.1246) construction
  line L773 (-90.886, 224.8248) -> (-90.6138, 224.1677) construction
  line L774 (-90.6138, 224.1677) -> (-90.5469, 223.8106) construction
  line L775 (-90.5469, 223.8106) -> (-90.5469, 223.4757) construction
  circle A146 centre (-88.5764, 237.6382) radius 1.25
  arc A147 (-100.5164, 218.0782) -> (-98.9289, 216.4907) centre (-98.9289, 218.0782) ccw
  line L776 (-98.9289, 216.4907) -> (-46.2275, 216.4907)
  arc A148 (97.1018, 216.039) -> (98.6893, 217.6265) centre (97.1018, 217.6265) ccw
  line L777 (93.9905, 222.332) -> (93.7184, 221.675) construction
  spline S24 degree 3 poles (94.0574, 223.024) (94.0574, 222.6891) (93.9905, 222.332) (93.7184, 221.675) (93.5132, 221.3751) (93.0397, 220.9015) (92.7397, 220.6962) (92.0826, 220.4239) (91.7253, 220.357) (91.0556, 220.357) (90.6984, 220.4239) (90.0412, 220.6961) (89.7412, 220.9014) (89.2677, 221.3751) (89.0625, 221.6749) (88.7903, 222.332) (88.7234, 222.6891) (88.7234, 223.3589) (88.7903, 223.716) (89.0625, 224.3731) (89.2677, 224.6729) (89.7412, 225.1466) (90.0412, 225.3519) (90.6984, 225.6241) (91.0556, 225.691) (91.7253, 225.691) (92.0826, 225.6241) (92.7397, 225.3518) (93.0397, 225.1465) (93.5132, 224.6729) (93.7184, 224.3731) (93.9905, 223.716) (94.0574, 223.3589) (94.0574, 223.024) knots -1.607821 -1.607821 -1.607821 -1.607821 -1.507361 -1.507361 -1.406901 -1.406901 -1.306377 -1.306377 -1.205854 -1.205854 -1.105342 -1.105342 -1.004829 -1.004829 -0.90437 -0.90437 -0.803911 -0.803911 -0.703451 -0.703451 -0.602992 -0.602992 -0.50248 -0.50248 -0.401967 -0.401967 -0.301444 -0.301444 -0.200921 -0.200921 -0.10046 -0.10046 0 0 0 0
  line L778 (94.0574, 223.024) -> (94.0574, 222.6891) construction
  line L779 (94.0574, 222.6891) -> (93.9905, 222.332) construction
  line L780 (93.7184, 221.675) -> (93.5132, 221.3751) construction
  line L781 (93.5132, 221.3751) -> (93.0397, 220.9015) construction
  line L782 (93.0397, 220.9015) -> (92.7397, 220.6962) construction
  line L783 (92.7397, 220.6962) -> (92.0826, 220.4239) construction
  line L784 (92.0826, 220.4239) -> (91.7253, 220.357) construction
  line L785 (91.7253, 220.357) -> (91.0556, 220.357) construction
  line L786 (91.0556, 220.357) -> (90.6984, 220.4239) construction
  line L787 (90.6984, 220.4239) -> (90.0412, 220.6961) construction
  line L788 (90.0412, 220.6961) -> (89.7412, 220.9014) construction
  line L789 (89.7412, 220.9014) -> (89.2677, 221.3751) construction
  line L790 (89.2677, 221.3751) -> (89.0625, 221.6749) construction
  line L791 (89.0625, 221.6749) -> (88.7903, 222.332) construction
  line L792 (88.7903, 222.332) -> (88.7234, 222.6891) construction
  line L793 (88.7234, 222.6891) -> (88.7234, 223.3589) construction
  line L794 (88.7234, 223.3589) -> (88.7903, 223.716) construction
  line L795 (88.7903, 223.716) -> (89.0625, 224.3731) construction
  line L796 (89.0625, 224.3731) -> (89.2677, 224.6729) construction
  line L797 (89.2677, 224.6729) -> (89.7412, 225.1466) construction
  line L798 (89.7412, 225.1466) -> (90.0412, 225.3519) construction
  line L799 (90.0412, 225.3519) -> (90.6984, 225.6241) construction
  line L800 (90.6984, 225.6241) -> (91.0556, 225.691) construction
  line L801 (91.0556, 225.691) -> (91.7253, 225.691) construction
  line L802 (91.7253, 225.691) -> (92.0826, 225.6241) construction
  line L803 (92.0826, 225.6241) -> (92.7397, 225.3518) construction
  line L804 (92.7397, 225.3518) -> (93.0397, 225.1465) construction
  line L805 (93.0397, 225.1465) -> (93.5132, 224.6729) construction
  line L806 (93.5132, 224.6729) -> (93.7184, 224.3731) construction
  line L807 (93.7184, 224.3731) -> (93.9905, 223.716) construction
  line L808 (93.9905, 223.716) -> (94.0574, 223.3589) construction
  line L809 (94.0574, 223.3589) -> (94.0574, 223.024) construction
  arc A149 (73.7529, 238.1865) -> (75.7529, 238.1865) centre (74.7529, 238.1865) ccw
  arc A150 (65.7529, 238.1865) -> (67.7529, 238.1865) centre (66.7529, 238.1865) ccw
  arc A151 (57.7529, 238.1865) -> (59.7529, 238.1865) centre (58.7529, 238.1865) ccw
  arc A152 (81.7529, 238.1865) -> (83.7529, 238.1865) centre (82.7529, 238.1865) ccw
  line L810 (44.4004, 216.039) -> (97.1018, 216.039)
  arc A153 (61.7529, 238.1865) -> (63.7529, 238.1865) centre (62.7529, 238.1865) ccw
  circle A154 centre (54.7529, 237.1865) radius 1.25
  line L811 (52.7824, 223.3589) -> (52.7824, 223.024) construction
  spline S25 degree 3 poles (52.7824, 223.024) (52.7824, 222.6891) (52.7155, 222.332) (52.4434, 221.6749) (52.2382, 221.3751) (51.7646, 220.9014) (51.4647, 220.6961) (50.8075, 220.4239) (50.4503, 220.357) (49.7805, 220.357) (49.4233, 220.4239) (48.7661, 220.6962) (48.4662, 220.9015) (47.9927, 221.3751) (47.7875, 221.675) (47.5154, 222.332) (47.4484, 222.6891) (47.4484, 223.3589) (47.5154, 223.716) (47.7875, 224.3731) (47.9927, 224.6729) (48.4662, 225.1465) (48.7661, 225.3518) (49.4233, 225.6241) (49.7805, 225.691) (50.4503, 225.691) (50.8075, 225.6241) (51.4647, 225.3519) (51.7646, 225.1466) (52.2382, 224.6729) (52.4434, 224.3731) (52.7155, 223.716) (52.7824, 223.3589) (52.7824, 223.024) knots -1.607821 -1.607821 -1.607821 -1.607821 -1.507362 -1.507362 -1.406903 -1.406903 -1.30639 -1.30639 -1.205878 -1.205878 -1.105355 -1.105355 -1.004831 -1.004831 -0.904371 -0.904371 -0.803911 -0.803911 -0.70345 -0.70345 -0.60299 -0.60299 -0.502467 -0.502467 -0.401943 -0.401943 -0.301431 -0.301431 -0.200918 -0.200918 -0.100459 -0.100459 0 0 0 0
  line L812 (52.7824, 223.024) -> (52.7824, 222.6891) construction
  line L813 (52.7824, 222.6891) -> (52.7155, 222.332) construction
  line L814 (52.7155, 222.332) -> (52.4434, 221.6749) construction
  line L815 (52.4434, 221.6749) -> (52.2382, 221.3751) construction
  line L816 (52.2382, 221.3751) -> (51.7646, 220.9014) construction
  line L817 (51.7646, 220.9014) -> (51.4647, 220.6961) construction
  line L818 (51.4647, 220.6961) -> (50.8075, 220.4239) construction
  line L819 (50.8075, 220.4239) -> (50.4503, 220.357) construction
  line L820 (50.4503, 220.357) -> (49.7805, 220.357) construction
  line L821 (49.7805, 220.357) -> (49.4233, 220.4239) construction
  line L822 (49.4233, 220.4239) -> (48.7661, 220.6962) construction
  line L823 (48.7661, 220.6962) -> (48.4662, 220.9015) construction
  line L824 (48.4662, 220.9015) -> (47.9927, 221.3751) construction
  line L825 (47.9927, 221.3751) -> (47.7875, 221.675) construction
  line L826 (47.7875, 221.675) -> (47.5154, 222.332) construction
  line L827 (47.5154, 222.332) -> (47.4484, 222.6891) construction
  line L828 (47.4484, 222.6891) -> (47.4484, 223.3589) construction
  line L829 (47.4484, 223.3589) -> (47.5154, 223.716) construction
  line L830 (47.5154, 223.716) -> (47.7875, 224.3731) construction
  line L831 (47.7875, 224.3731) -> (47.9927, 224.6729) construction
  line L832 (47.9927, 224.6729) -> (48.4662, 225.1465) construction
  line L833 (48.4662, 225.1465) -> (48.7661, 225.3518) construction
  line L834 (48.7661, 225.3518) -> (49.4233, 225.6241) construction
  line L835 (49.4233, 225.6241) -> (49.7805, 225.691) construction
  line L836 (49.7805, 225.691) -> (50.4503, 225.691) construction
  line L837 (50.4503, 225.691) -> (50.8075, 225.6241) construction
  line L838 (50.8075, 225.6241) -> (51.4647, 225.3519) construction
  line L839 (51.4647, 225.3519) -> (51.7646, 225.1466) construction
  line L840 (51.7646, 225.1466) -> (52.2382, 224.6729) construction
  line L841 (52.2382, 224.6729) -> (52.4434, 224.3731) construction
  line L842 (52.4434, 224.3731) -> (52.7155, 223.716) construction
  line L843 (52.7155, 223.716) -> (52.7824, 223.3589) construction
  arc A155 (42.8129, 217.6265) -> (44.4004, 216.039) centre (44.4004, 217.6265) ccw
  arc A156 (69.7529, 238.1865) -> (71.7529, 238.1865) centre (70.7529, 238.1865) ccw
  arc A157 (77.7529, 238.1865) -> (79.7529, 238.1865) centre (78.7529, 238.1865) ccw
  circle A158 centre (86.7529, 237.1865) radius 1.25
  line L844 (69.7529, 238.1865) -> (69.7529, 277.269)
  line L845 (71.7529, 277.269) -> (71.7529, 238.1865)
  line L846 (83.7529, 275.0908) -> (83.7529, 238.1865)
  line L847 (57.7529, 238.1865) -> (57.7529, 275.0908)
  line L848 (73.7529, 238.1865) -> (73.7529, 277.269)
  line L849 (67.7529, 277.269) -> (67.7529, 238.1865)
  line L850 (75.7529, 277.269) -> (75.7529, 238.1865)
  line L851 (77.7529, 238.1865) -> (77.7529, 277.269)
  line L852 (63.7529, 277.269) -> (63.7529, 238.1865)
  line L853 (79.7529, 277.269) -> (79.7529, 238.1865)
  line L854 (61.7529, 238.1865) -> (61.7529, 277.269)
  line L855 (81.7529, 238.1865) -> (81.7529, 277.269)
  line L856 (59.7529, 277.269) -> (59.7529, 238.1865)
  line L857 (98.6893, 217.6265) -> (98.6893, 291.9215)
  line L858 (42.8129, 292.5565) -> (42.8129, 217.6265)
  line L859 (65.7529, 238.1865) -> (65.7529, 277.269)
  line L860 (48.7661, 284.1962) -> (48.4662, 284.4015) construction
  spline S26 degree 3 poles (52.7824, 286.524) (52.7824, 286.1891) (52.7155, 285.832) (52.4434, 285.1749) (52.2382, 284.8751) (51.7646, 284.4014) (51.4647, 284.1961) (50.8075, 283.9239) (50.4503, 283.857) (49.7805, 283.857) (49.4233, 283.9239) (48.7661, 284.1962) (48.4662, 284.4015) (47.9927, 284.8751) (47.7875, 285.175) (47.5154, 285.832) (47.4484, 286.1891) (47.4484, 286.8589) (47.5154, 287.216) (47.7875, 287.8731) (47.9927, 288.1729) (48.4662, 288.6465) (48.7661, 288.8518) (49.4233, 289.1241) (49.7805, 289.191) (50.4503, 289.191) (50.8075, 289.1241) (51.4647, 288.8519) (51.7646, 288.6466) (52.2382, 288.1729) (52.4434, 287.8731) (52.7155, 287.216) (52.7824, 286.8589) (52.7824, 286.524) knots -1.607821 -1.607821 -1.607821 -1.607821 -1.507362 -1.507362 -1.406903 -1.406903 -1.30639 -1.30639 -1.205878 -1.205878 -1.105355 -1.105355 -1.004831 -1.004831 -0.904371 -0.904371 -0.803911 -0.803911 -0.70345 -0.70345 -0.60299 -0.60299 -0.502467 -0.502467 -0.401943 -0.401943 -0.301431 -0.301431 -0.200918 -0.200918 -0.100459 -0.100459 0 0 0 0
  line L861 (52.7824, 286.524) -> (52.7824, 286.1891) construction
  line L862 (52.7824, 286.1891) -> (52.7155, 285.832) construction
  line L863 (52.7155, 285.832) -> (52.4434, 285.1749) construction
  line L864 (52.4434, 285.1749) -> (52.2382, 284.8751) construction
  line L865 (52.2382, 284.8751) -> (51.7646, 284.4014) construction
  line L866 (51.7646, 284.4014) -> (51.4647, 284.1961) construction
  line L867 (51.4647, 284.1961) -> (50.8075, 283.9239) construction
  line L868 (50.8075, 283.9239) -> (50.4503, 283.857) construction
  line L869 (50.4503, 283.857) -> (49.7805, 283.857) construction
  line L870 (49.7805, 283.857) -> (49.4233, 283.9239) construction
  line L871 (49.4233, 283.9239) -> (48.7661, 284.1962) construction
  line L872 (48.4662, 284.4015) -> (47.9927, 284.8751) construction
  line L873 (47.9927, 284.8751) -> (47.7875, 285.175) construction
  line L874 (47.7875, 285.175) -> (47.5154, 285.832) construction
  line L875 (47.5154, 285.832) -> (47.4484, 286.1891) construction
  line L876 (47.4484, 286.1891) -> (47.4484, 286.8589) construction
  line L877 (47.4484, 286.8589) -> (47.5154, 287.216) construction
  line L878 (47.5154, 287.216) -> (47.7875, 287.8731) construction
  line L879 (47.7875, 287.8731) -> (47.9927, 288.1729) construction
  line L880 (47.9927, 288.1729) -> (48.4662, 288.6465) construction
  line L881 (48.4662, 288.6465) -> (48.7661, 288.8518) construction
  line L882 (48.7661, 288.8518) -> (49.4233, 289.1241) construction
  line L883 (49.4233, 289.1241) -> (49.7805, 289.191) construction
  line L884 (49.7805, 289.191) -> (50.4503, 289.191) construction
  line L885 (50.4503, 289.191) -> (50.8075, 289.1241) construction
  line L886 (50.8075, 289.1241) -> (51.4647, 288.8519) construction
  line L887 (51.4647, 288.8519) -> (51.7646, 288.6466) construction
  line L888 (51.7646, 288.6466) -> (52.2382, 288.1729) construction
  line L889 (52.2382, 288.1729) -> (52.4434, 287.8731) construction
  line L890 (52.4434, 287.8731) -> (52.7155, 287.216) construction
  line L891 (52.7155, 287.216) -> (52.7824, 286.8589) construction
  line L892 (52.7824, 286.8589) -> (52.7824, 286.524) construction
  line L893 (50.4329, 294.144) -> (44.4004, 294.144)
  arc A159 (44.4004, 294.144) -> (42.8129, 292.5565) centre (44.4004, 292.5565) ccw
  line L894 (56.7829, 285.836) -> (56.7829, 287.794)
  arc A160 (56.7829, 287.794) -> (50.4329, 294.144) centre (50.4329, 287.794) ccw
  arc A161 (84.2379, 280.4634) -> (84.7229, 285.836) centre (54.7229, 285.836) ccw
  line L895 (84.7229, 287.159) -> (84.7229, 285.836)
  circle A162 centre (86.7529, 269.1865) radius 1.25
  arc A163 (65.7529, 277.269) -> (63.7529, 277.269) centre (64.7529, 277.269) ccw
  arc A164 (69.7529, 277.269) -> (67.7529, 277.269) centre (68.7529, 277.269) ccw
  arc A165 (73.7529, 277.269) -> (71.7529, 277.269) centre (72.7529, 277.269) ccw
  arc A166 (77.7529, 277.269) -> (75.7529, 277.269) centre (76.7529, 277.269) ccw
  arc A167 (81.7529, 277.269) -> (79.7529, 277.269) centre (80.7529, 277.269) ccw
  arc A168 (84.2379, 280.4634) -> (83.7529, 275.0908) centre (113.7529, 275.0908) ccw
  line L896 (94.0574, 286.1891) -> (93.9905, 285.832) construction
  spline S27 degree 3 poles (94.0574, 286.524) (94.0574, 286.1891) (93.9905, 285.832) (93.7184, 285.175) (93.5132, 284.8751) (93.0397, 284.4015) (92.7397, 284.1962) (92.0826, 283.9239) (91.7253, 283.857) (91.0556, 283.857) (90.6984, 283.9239) (90.0412, 284.1961) (89.7412, 284.4014) (89.2677, 284.8751) (89.0625, 285.1749) (88.7903, 285.832) (88.7234, 286.1891) (88.7234, 286.8589) (88.7903, 287.216) (89.0625, 287.8731) (89.2677, 288.1729) (89.7412, 288.6466) (90.0412, 288.8519) (90.6984, 289.1241) (91.0556, 289.191) (91.7253, 289.191) (92.0826, 289.1241) (92.7397, 288.8518) (93.0397, 288.6465) (93.5132, 288.1729) (93.7184, 287.8731) (93.9905, 287.216) (94.0574, 286.8589) (94.0574, 286.524) knots -1.607821 -1.607821 -1.607821 -1.607821 -1.507361 -1.507361 -1.406901 -1.406901 -1.306377 -1.306377 -1.205854 -1.205854 -1.105342 -1.105342 -1.004829 -1.004829 -0.90437 -0.90437 -0.803911 -0.803911 -0.703451 -0.703451 -0.602992 -0.602992 -0.50248 -0.50248 -0.401967 -0.401967 -0.301444 -0.301444 -0.200921 -0.200921 -0.10046 -0.10046 0 0 0 0
  line L897 (94.0574, 286.524) -> (94.0574, 286.1891) construction
  line L898 (93.9905, 285.832) -> (93.7184, 285.175) construction
  line L899 (93.7184, 285.175) -> (93.5132, 284.8751) construction
  line L900 (93.5132, 284.8751) -> (93.0397, 284.4015) construction
  line L901 (93.0397, 284.4015) -> (92.7397, 284.1962) construction
  line L902 (92.7397, 284.1962) -> (92.0826, 283.9239) construction
  line L903 (92.0826, 283.9239) -> (91.7253, 283.857) construction
  line L904 (91.7253, 283.857) -> (91.0556, 283.857) construction
  line L905 (91.0556, 283.857) -> (90.6984, 283.9239) construction
  line L906 (90.6984, 283.9239) -> (90.0412, 284.1961) construction
  line L907 (90.0412, 284.1961) -> (89.7412, 284.4014) construction
  line L908 (89.7412, 284.4014) -> (89.2677, 284.8751) construction
  line L909 (89.2677, 284.8751) -> (89.0625, 285.1749) construction
  line L910 (89.0625, 285.1749) -> (88.7903, 285.832) construction
  line L911 (88.7903, 285.832) -> (88.7234, 286.1891) construction
  line L912 (88.7234, 286.1891) -> (88.7234, 286.8589) construction
  line L913 (88.7234, 286.8589) -> (88.7903, 287.216) construction
  line L914 (88.7903, 287.216) -> (89.0625, 287.8731) construction